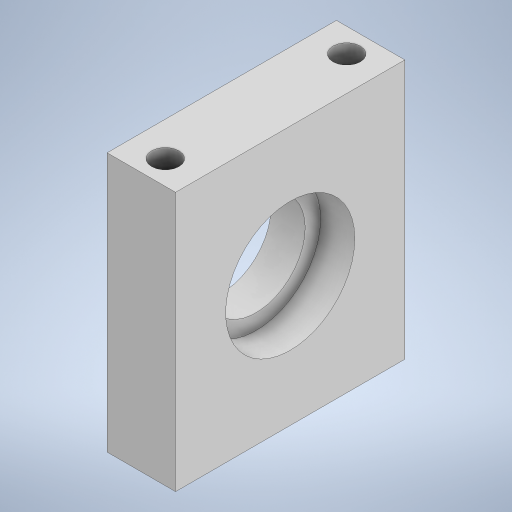
# Autodesk Inventor part: Differential mount
Saved by Autodesk Inventor 2023 (Build 270158000, 158)
## iProperties
Created: 2023-05-22
Part Number: Differential mount
Material: Типовые
Document SubType Name: Modeling
Designer: ivanc
Density: 1 g/cm^3
Appearance: По умолчанию
Author: ivanc
Autodesk Inventor part; units mm, degrees
ref_plane "YZ Plane" through (0, 0, 0) normal (1, 0, 0) x (0, 1, 0)
ref_plane "XZ Plane" through (0, 0, 0) normal (0, 1, 0) x (-1, 0, 0)
ref_plane "XY Plane" through (0, 0, 0) normal (0, 0, 1) x (1, 0, 0)
sketch "Эскиз1" plane through (0, 0, 0) normal (1, 0, 0) x (0, 1, 0)
  line L0 (-15.15, 13.4) -> (15.15, 13.4)
  line L1 (15.15, 13.4) -> (15.15, -13.4)
  line L2 (15.15, -13.4) -> (-15.15, -13.4)
  line L3 (-15.15, -13.4) -> (-15.15, 13.4)
  line L4 (-15.15, 13.4) -> (15.15, -13.4) construction
  line L5 (15.15, 13.4) -> (-15.15, -13.4) construction
  point P0 (0, 0)
  dimension "d0" = 30.3
  dimension "d1" = 26.8
  constraints: 12 end point, 2 midpoint, 2 parallel, 1 horizontal, 1 perpendicular
  measures "d0" distance of L1.end L2.end
  measures "d1" distance of L0.end L1.end
extrude "Выдавливание1" add sketch "Эскиз1" along normal blind 8
sketch "Эскиз2" plane through (0, 15.15, 13.4) normal (0, 1, 0) x (1, 0, 0)
  line L0 (4, 2.8) -> (4, 24)
  line L1 (0, 13.4) -> (8, 13.4)
  line L2 (0, 26.8) -> (0, 0) projected
  line L3 (8, 26.8) -> (8, 0) projected
  point P0 (0, 13.4)
  point P1 (4, 13.4)
  dimension "d4" = 21.2
  constraints: 4 end point, 4 midpoint, 1 perpendicular
  measures "d4" distance of L0.start L0.end
hole "Отверстие1" at (4, 15.15, 10.6) at (4, 15.15, -10.6) direction (0, -1, 0) diameter 3.2 end through all
sketch "Эскиз3" plane through (8, 0, 0) normal (1, 0, 0) x (0, 0, -1)
  line L0 (13.4, 15.15) -> (-13.4, 15.15) projected
  line L1 (-13.4, -15.15) -> (13.4, -15.15) projected
  line L2 (-13.4, 15.15) -> (13.4, -15.15)
  circle A0 centre (0, 0) radius 5.75
  dimension "d12" = 11.5
  constraints: 2 end point, 1 centre point, 1 coincident
  measures "d12" diameter of A0
extrude "Выдавливание2" cut sketch "Эскиз3" against normal through all
sketch "Эскиз4" plane through (8, 0, 0) normal (1, 0, 0) x (0, 0, -1)
  circle A0 centre (0, 0) radius 5.75 projected
  circle A1 centre (0, 0) radius 7.55
  dimension "d15" = 15.1
  constraints: 1 centre point, 1 concentric
  measures "d15" diameter of A1
extrude "Выдавливание3" cut sketch "Эскиз4" against normal blind 4 contours A0 | A1
